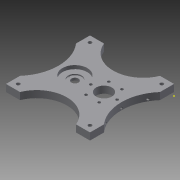
# Autodesk Inventor part: Traveler
Saved by Autodesk Inventor 2015 (Build 190159000, 159)
## iProperties
Created: 2015-01-23
Part Number: Traveler
Material: Generic
Document SubType Name: Modeling
Designer: chappelled
Density: 1 g/cm^3
Appearance: Default
Author: chappelled
Autodesk Inventor part; units mm, degrees
ref_plane "YZ Plane" through (0, 0, 0) normal (1, 0, 0) x (0, 1, 0)
ref_plane "XZ Plane" through (0, 0, 0) normal (0, 1, 0) x (-1, 0, 0)
sketch "Sketch1" plane through (0, 0, 0) normal (0, 1, 0) x (-1, 0, 0)
  line L0 (0, 0) -> (152.4, 0)
  line L1 (152.4, 0) -> (152.4, 152.4)
  line L2 (152.4, 152.4) -> (0, 152.4)
  line L3 (0, 152.4) -> (0, 0)
  dimension "d0" = 152.4
  dimension "d1" = 152.4
  constraints: 8 end point, 2 parallel, 1 horizontal, 1 perpendicular
  measures "d0" distance of L2.end L1.end
  measures "d1" distance of L1.end L0.end
extrude "Extrusion1" add sketch "Sketch1" along normal blind 12.7
hole "Hole1" at (-103.5558, 12.7, 76.2) direction (0, -1, 0) diameter 12.7 end through all
hole "Hole2" at (-50.8, 12.7, 76.2) direction (0, -1, 0) diameter 28.575 end through all
hole "Hole3" at (38.1, 0, 58.6994) direction (0, 1, 0) diameter 4.5 end through all countersink diameter 9.525 countersink angle 82
pattern_circular "Circular Pattern1" count 4 over 360 about axis through (-103.5558, -203.2, 76.2) along (0, 1, 0) of "Hole3"
sketch "Sketch4" plane through (0, 12.7, 0) normal (0, 1, 0) x (1, 0, 0)
  circle A0 centre (-103.5558, -76.2) radius 6.35 projected
  circle A1 centre (-103.5558, -76.2) radius 12.0332
  dimension "d41" = 24.0665
  constraints: 1 centre point, 1 coincident
  measures "d41" diameter of A1
sketch "Sketch5" plane through (0, 12.7, 0) normal (0, 1, 0) x (1, 0, 0)
  circle A0 centre (-50.8, -76.2) radius 14.2875 projected
  circle A1 centre (-103.5558, -76.2) radius 6.35 projected
  line L0 (0, 0) -> (-152.4, 0) projected
  line L1 (-152.4, 0) -> (-152.4, -152.4) projected
  line L2 (-152.4, -152.4) -> (0, -152.4) projected
  line L3 (0, -152.4) -> (0, 0) projected
  circle A2 centre (-103.5558, -76.2) radius 22.5425
  dimension "d42" = 45.085
  constraints: 1 centre point, 1 coincident
  measures "d42" diameter of A2
extrude "Extrusion4" add sketch "Sketch5" along normal blind 6.35 contours L3 L2 L1 L0
extrude "Extrusion5" cut sketch "Sketch4" against normal blind 2.032
hole "Hole4" at (-26.9748, 0, 76.2) direction (0, 1, 0) diameter 5.08 end through all countersink diameter 9.525 countersink angle 82
pattern_circular "Circular Pattern2" count 6 over 360 about axis through (-50.8, 19.05, 76.2) along (0, -1, 0) of "Hole4"
hole "Hole5" at (0, 9.525, 114.3) direction (-1, 0, 0) diameter 3.9624 depth 38.1 tip angle 118 thread size "10-32 UNF" class "2B" standard "ANSI Unified Screw Threads"
pattern_linear "Rectangular Pattern1" count 3 spacing 38.1 along (0, 0, -1) of "Hole5"
ref_plane "Work Plane1" through (-76.2, 0, 0) normal (-1, 0, 0) x (0, 0, 1)
mirror "Mirror1" about plane through (-76.2, 0, 0) normal (-1, 0, 0) of "Hole5", "Rectangular Pattern1"
sketch "Sketch6" plane through (0, 19.05, 0) normal (0, 1, 0) x (1, 0, 0)
  circle A0 centre (-11.1125, -11.1125) radius 3.175
  circle A1 centre (-11.1125, -141.2875) radius 3.175
  circle A2 centre (-141.2875, -11.1125) radius 3.175
  circle A3 centre (-141.2875, -141.2875) radius 3.175
  line L0 (0, 0) -> (-152.4, 0) projected
  line L1 (0, -152.4) -> (0, 0) projected
  line L2 (-152.4, -152.4) -> (0, -152.4) projected
  line L3 (-152.4, 0) -> (-152.4, -152.4) projected
  dimension "d78" = 6.35
  dimension "d79" = 6.35
  dimension "d80" = 6.35
  dimension "d81" = 6.35
  dimension "d82" = 11.1125
  dimension "d83" = 11.1125
  dimension "d84" = 11.1125
  dimension "d85" = 11.1125
  dimension "d86" = 11.1125
  dimension "d87" = 11.1125
  dimension "d88" = 11.1125
  dimension "d89" = 11.1125
  constraints: 4 centre point
  measures "d78" diameter of A0
  measures "d79" diameter of A1
  measures "d80" diameter of A2
  measures "d81" diameter of A3
  measures "d82" distance from line of L0 A0.centre
  measures "d83" distance from line of L1 A0.centre
  measures "d84" distance from line of L2 A1.centre
  measures "d85" distance from line of L1 A1.centre
  measures "d86" distance from line of L2 A3.centre
  measures "d87" distance from line of L3 A3.centre
  measures "d88" distance from line of A2.centre L0
  measures "d89" distance from line of L3 A2.centre
extrude "Extrusion6" cut sketch "Sketch6" against normal blind 25.4 contours A0 | A1 | A2 | A3
sketch "Sketch7" plane through (0, 19.05, 0) normal (0, 1, 0) x (1, 0, 0)
  line L0 (0, 0) -> (-152.4, 0) projected
  line L1 (-152.4, 0) -> (-152.4, -152.4) projected
  line L2 (0, -152.4) -> (0, 0) projected
  arc A0 (-127, 0) -> (-25.4, 0) centre (-76.2, 20.5322) ccw
  line L3 (-127, 0) -> (-25.4, 0)
  line L4 (-152.4, -152.4) -> (0, -152.4) projected
  arc A1 (-25.4, -152.4) -> (-127, -152.4) centre (-76.2, -172.9198) ccw
  line L5 (-152.4, 0) -> (-152.4, -152.4) projected
  line L6 (0, -152.4) -> (0, 0) projected
  arc A2 (-152.4, -127) -> (-152.4, -25.4) centre (-210.6083, -76.2) ccw
  arc A3 (0, -25.4) -> (0, -127) centre (58.2083, -76.2) ccw
  line L7 (0, -25.4) -> (0, -127)
  line L8 (-152.4, -25.4) -> (-152.4, -127)
  line L9 (-127, -152.4) -> (-25.4, -152.4)
  line L10 (-152.4, -152.4) -> (0, -152.4) projected
  dimension "d92" = 25.4
  dimension "d93" = 25.4
  dimension "d94" = 25.4
  dimension "d95" = 25.4
  dimension "d97" = 54.7878
  dimension "d98" = 25.4
  dimension "d99" = 25.4
  dimension "d100" = 25.4
  dimension "d101" = 25.4
  constraints: 8 end point, 8 point on circle, 8 point on line, 4 centre point, 3 collinear, 1 parallel
  measures "d92" distance from line of L1 L3.start
  measures "d93" distance from line of L2 L3.end
  measures "d94" distance from line of L9.start L1
  measures "d95" distance from line of L2 L9.end
  measures "d97" radius of A1
  measures "d98" distance from line of L8.start L0
  measures "d99" distance from line of L7.start L0
  measures "d100" distance from line of L7.end L4
  measures "d101" distance from line of L8.end L4
extrude "Extrusion7" cut sketch "Sketch7" against normal blind 25.4 contours A0 L0 | L2 A3 | A2 L1 | L4 A1
sketch "Sketch8" plane through (0, 0, 0) normal (0, -1, 0) x (1, 0, 0)
  point P0 (0, 0)
sketch "Sketch9" plane through (0, 0, 0) normal (0, -1, 0) x (1, 0, 0)
  line L0 (-152.4, 25.4) -> (-152.4, 0)
  line L1 (-152.4, 0) -> (-152.4, 25.4) projected
  line L2 (-152.4, 0) -> (-127, 0)
  line L3 (-127, 0) -> (-152.4, 0) projected
  line L4 (-127, 0) -> (0, 0)
  line L5 (0, 0) -> (-25.4, 0) projected
  line L6 (0, 0) -> (0, 25.4)
  line L7 (0, 25.4) -> (0, 0) projected
  line L8 (0, 25.4) -> (0, 127)
  line L9 (0, 127) -> (0, 152.4)
  line L10 (0, 152.4) -> (0, 127) projected
  line L11 (0, 152.4) -> (-25.4, 152.4)
  line L12 (-25.4, 152.4) -> (0, 152.4) projected
  line L13 (-25.4, 152.4) -> (-127, 152.4)
  line L14 (-127, 152.4) -> (-152.4, 152.4)
  line L15 (-152.4, 152.4) -> (-127, 152.4) projected
  line L16 (-152.4, 152.4) -> (-152.4, 127)
  line L17 (-152.4, 127) -> (-152.4, 152.4) projected
  line L18 (-152.4, 127) -> (-152.4, 25.4)
  arc A0 (-152.4, 25.4) -> (-152.4, 127) centre (-210.6083, 76.2) ccw
  arc A1 (-152.4, 25.4) -> (-152.4, 127) centre (-210.6083, 76.2) ccw projected
  arc A2 (-127, 152.4) -> (-25.4, 152.4) centre (-76.2, 172.9198) ccw
  arc A3 (-25.4, 0) -> (-127, 0) centre (-76.2, -20.5322) ccw
  arc A4 (-25.4, 0) -> (-127, 0) centre (-76.2, -20.5322) ccw projected
  arc A5 (0, 127) -> (0, 25.4) centre (58.2083, 76.2) ccw
  constraints: 22 end point, 10 collinear, 8 point on circle, 4 centre point, 2 concentric, 1 point on line
extrude "Extrusion8" cut sketch "Sketch9" against normal blind 6.35 contours A0 L16 L14 A2 L11 L9 A5 L6 L4 A3 L2 L0
body "Solid1"
